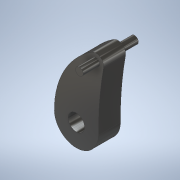
# Autodesk Inventor part: Part33
Saved by Autodesk Inventor 2021 (Build 250183000, 183)
## iProperties
Created: 2020-11-16
Part Number: Part33
Material: Liga de Nickel-Copper 400
Document SubType Name: Modeling
Designer: Lucas Moura
Density: 8.83 g/cm^3
Appearance: Cromado - Preto polido
Author: Lucas Moura
Autodesk Inventor part; units mm, degrees
ref_plane "YZ Plane" through (0, 0, 0) normal (1, 0, 0) x (0, 1, 0)
ref_plane "XZ Plane" through (0, 0, 0) normal (0, 1, 0) x (-1, 0, 0)
ref_plane "XY Plane" through (0, 0, 0) normal (0, 0, 1) x (1, 0, 0)
sketch "Sketch1" plane through (0, 0, 0) normal (0, 0, 1) x (1, 0, 0)
  line L0 (0, 0) -> (20, 0) construction
  line L1 (20, 0) -> (20, 20) construction
  line L2 (20, 20) -> (0, 20) construction
  line L3 (0, 20) -> (0, 0) construction
  circle A0 centre (7.9375, 4.7625) radius 2
  circle A1 centre (7.9375, 4.7625) radius 0.75
  arc A2 (10.691, 11.6731) -> (5.9394, 4.676) centre (13.3396, 4.7625) ccw
  arc A3 (10.691, 11.6731) -> (9.9375, 4.7625) centre (38.5656, 5.1375) ccw
  dimension "d0" = 20
  dimension "d1" = 20
  dimension "d2" = 4
  dimension "d3" = 1.5
  constraints: 8 end point, 6 point on circle, 4 centre point, 2 parallel, 1 coincident, 1 horizontal, 1 perpendicular
  measures "d0" distance of L1.end L2.end
  measures "d1" distance of L0.end L1.end
  measures "d2" diameter of A0
  measures "d3" diameter of A1
extrude "Extrusion1" add sketch "Sketch1" along normal blind 2 contours A0 A2 A3
fillet "Fillet2" radius 0.7 1 edges at (10.691, 11.6731, 1)
sketch "Sketch2" plane through (0, 0, 2) normal (0, 0, 1) x (1, 0, 0)
  arc A0 (5.9394, 4.676) -> (9.9375, 4.7625) centre (7.9375, 4.7625) ccw projected
  circle A1 centre (7.9375, 4.7625) radius 0.75 projected
  arc A2 (10.3988, 10.2697) -> (9.9375, 4.7625) centre (38.5656, 5.1375) ccw projected
  arc A3 (9.331, 10.9836) -> (5.9394, 4.676) centre (13.3396, 4.7625) ccw projected
  arc A4 (10.3988, 10.2697) -> (9.331, 10.9836) centre (9.7101, 10.3952) ccw projected
  circle A5 centre (9.7101, 10.3952) radius 0.35
  point P0 (0, 0)
  dimension "d16" = 0.7
  constraints: 1 centre point, 1 coincident
  measures "d16" diameter of A5
extrude "Extrusion2" add sketch "Sketch2" along normal blind 1.5 contours A5
sketch "Sketch3" plane through (0, 0, 0) normal (0, 0, -1) x (-1, 0, 0)
  arc A0 (-9.9375, 4.7625) -> (-5.9394, 4.676) centre (-7.9375, 4.7625) ccw projected
  circle A1 centre (-7.9375, 4.7625) radius 0.75 projected
  arc A2 (-5.9394, 4.676) -> (-9.331, 10.9836) centre (-13.3396, 4.7625) ccw projected
  arc A3 (-9.9375, 4.7625) -> (-10.3988, 10.2697) centre (-38.5656, 5.1375) ccw projected
  arc A4 (-9.331, 10.9836) -> (-10.3988, 10.2697) centre (-9.7101, 10.3952) ccw projected
  circle A5 centre (-9.7101, 10.3952) radius 0.35
  point P0 (0, 0)
  dimension "d17" = 0.7
  constraints: 1 centre point, 1 coincident
  measures "d17" diameter of A5
extrude "Extrusion3" add sketch "Sketch3" along normal blind 1.5 contours A5
body "Solid1"
